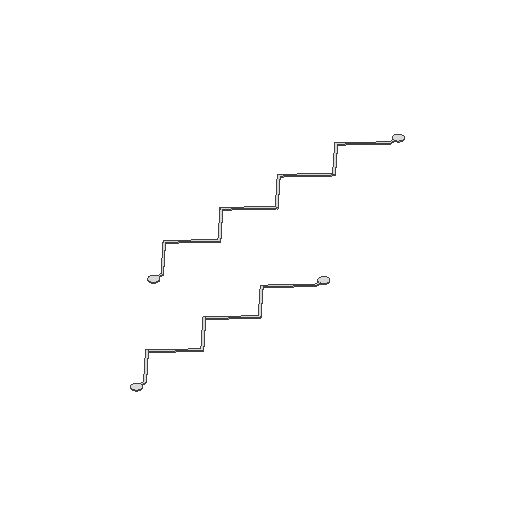
# Autodesk Inventor part: Serpentine
Saved by Autodesk Inventor 2025.4 (Build 294407000, 407)
## iProperties
Created: 2026-04-28
Part Number: Serpentine
Material: Generic
Document SubType Name: Modeling
Designer: gdira
Density: 1 g/cm^3
Appearance: Default
Author: gdira
Autodesk Inventor part; units mm, degrees
ref_plane "YZ Plane" through (0, 0, 0) normal (1, 0, 0) x (0, 1, 0)
ref_plane "XZ Plane" through (0, 0, 0) normal (0, 1, 0) x (-1, 0, 0)
ref_plane "XY Plane" through (0, 0, 0) normal (0, 0, 1) x (1, 0, 0)
sketch "Sketch1" plane through (0, 0, 0) normal (0, 1, 0) x (-1, 0, 0)
  line L0 (15, -130) -> (0, -130)
  line L1 (1.2651, -65) -> (15, -65)
  line L2 (1.2609, -97.5) -> (15, -97.5)
  line L3 (13.5021, -113.8888) -> (-0.2581, -115.1476)
  line L4 (15, -65) -> (1.2651, -65)
  line L5 (13.4695, -81.25) -> (-0.2581, -79.8524)
  line L6 (14.8669, 0) -> (0.0022, 0)
  line L7 (1.2651, -32.5) -> (15, -32.5)
  line L8 (13.4697, -16.25) -> (-0.2581, -14.8524)
  line L9 (13.4697, -48.75) -> (-0.2581, -50.1476)
  line L10 (0, -129.7127) -> (15, -113.75)
  line L11 (15, -113.75) -> (14.2713, -113.0652)
  line L12 (13.5021, -113.8888) -> (-1, -129.3217)
  line L13 (-1, -129.3217) -> (-0.9978, -129.3238)
  line L14 (15, -113.75) -> (0.6282, -98.1807)
  line L15 (-0.2652, -97.5) -> (-1, -98.1783)
  line L16 (-1, -98.1783) -> (13.5021, -113.8888)
  line L17 (14.2652, -114.4283) -> (15, -113.75)
  line L18 (-1, -98.1783) -> (14.102, -81.9307)
  line L19 (15, -81.25) -> (15.7325, -81.9308)
  line L20 (-0.2605, -98.8657) -> (-1, -98.1783)
  line L21 (15.7325, -81.9308) -> (0.6326, -65.6807)
  line L22 (-0.2652, -65) -> (-0.9978, -65.6807)
  line L23 (-0.9978, -65.6807) -> (14.102, -81.9307)
  line L24 (14.9999, -82.6115) -> (15.7325, -81.9308)
  line L25 (-0.9978, -65.6807) -> (14.1022, -49.4307)
  line L26 (15, -48.75) -> (15.7326, -49.4307)
  line L27 (15.7326, -49.4307) -> (0.6326, -65.6807)
  line L28 (-0.2652, -66.3614) -> (-0.9978, -65.6807)
  line L29 (15.7326, -49.4307) -> (0.6325, -33.1807)
  line L30 (-0.2652, -32.5) -> (-0.9978, -33.1807)
  line L31 (-0.9978, -33.1807) -> (14.1022, -49.4307)
  line L32 (15, -50.1114) -> (15.7326, -49.4307)
  line L33 (-0.9978, -33.1807) -> (14.1018, -16.9303)
  line L34 (14.8669, -16.3923) -> (15.5995, -17.073)
  line L35 (15.5995, -17.073) -> (0.6325, -33.1807)
  line L36 (-0.2652, -33.8614) -> (-0.9978, -33.1807)
  line L37 (15.5995, -17.073) -> (0.0022, -0.2878)
  line L38 (-0.9978, -0.6807) -> (14.1018, -16.9303)
  line L39 (15, -17.6114) -> (15.5995, -17.073)
  line L40 (-0.2652, -129.3217) -> (0, -129.3217)
  line L41 (0, -129.3217) -> (0, -131.8722)
  line L42 (-1, -131.8722) -> (-1, -129.3217)
  line L43 (0, -0.6807) -> (0.0022, -0.6807)
  line L44 (0.0022, -0.2878) -> (0.0022, 1.8698)
  line L45 (-0.9978, 1.8698) -> (-0.9978, -0.6807)
  arc A0 (0.0022, 1.8698) -> (-0.9978, 1.8698) centre (-0.4978, 4.3193) ccw
  arc A1 (-1, -131.8722) -> (0, -131.8722) centre (-0.5, -134.3217) ccw
  line L46 (0, -134.3217) -> (-0.2652, -134.3217)
  line L47 (-0.9978, -134.3217) -> (-1, -134.3217)
  line L48 (15.7325, -81.9308) -> (0.6282, -98.1807)
  line L49 (-0.2581, -98.8631) -> (-0.2605, -98.8657)
  line L50 (15, -82.6114) -> (15, -130)
  line L51 (-0.2652, -97.5) -> (-0.2652, -66.3614)
  line L52 (15, -50.1114) -> (15, -81.25)
  line L53 (-0.2652, -65) -> (-0.2652, -33.8614)
  line L54 (-0.2652, -32.5) -> (-0.2652, -1.4691)
  line L55 (14.8669, 0) -> (14.8669, -16.3923)
  line L56 (15, -17.6114) -> (15, -48.75)
  line L57 (0.0022, 4.3193) -> (0, 4.3193)
  line L58 (-0.2581, -128.5323) -> (-0.2581, -98.8631)
  line L59 (-33.8119, -38.9953) -> (-48.8119, -38.9953)
  line L60 (-47.5468, 26.0047) -> (-33.8119, 26.0047)
  line L61 (-47.5509, -6.4953) -> (-33.8119, -6.4953)
  line L62 (-35.3097, -22.8842) -> (-49.07, -24.1429)
  line L63 (-33.8119, 26.0047) -> (-47.5468, 26.0047)
  line L64 (-35.3424, 9.7546) -> (-49.07, 11.1522)
  line L65 (-35.3422, 42.2547) -> (-49.07, 40.8571)
  line L66 (-48.8119, -38.708) -> (-33.8119, -22.7453)
  line L67 (-33.8119, -22.7453) -> (-34.5406, -22.0605)
  line L68 (-35.3097, -22.8842) -> (-49.8119, -38.317)
  line L69 (-49.8119, -38.317) -> (-49.8096, -38.3191)
  line L70 (-33.8119, -22.7453) -> (-48.1836, -7.176)
  line L71 (-49.0771, -6.4953) -> (-49.8119, -7.1736)
  line L72 (-49.8119, -7.1736) -> (-35.3097, -22.8842)
  line L73 (-34.5467, -23.4236) -> (-33.8119, -22.7453)
  line L74 (-49.8119, -7.1736) -> (-34.7099, 9.0739)
  line L75 (-33.8119, 9.7547) -> (-33.0794, 9.0739)
  line L76 (-49.0724, -7.861) -> (-49.8119, -7.1736)
  line L77 (-33.0794, 9.0739) -> (-48.1793, 25.324)
  line L78 (-49.0771, 26.0047) -> (-49.8096, 25.324)
  line L79 (-49.8096, 25.324) -> (-34.7099, 9.0739)
  line L80 (-33.812, 8.3932) -> (-33.0794, 9.0739)
  line L81 (-49.8096, 25.324) -> (-34.7096, 41.574)
  line L82 (-33.8119, 42.2547) -> (-33.0793, 41.574)
  line L83 (-33.0793, 41.574) -> (-48.1793, 25.324)
  line L84 (-49.0771, 24.6433) -> (-49.8096, 25.324)
  line L85 (-33.0793, 41.574) -> (-48.1793, 57.824)
  line L86 (-49.8096, 57.8239) -> (-34.7096, 41.574)
  line L87 (-33.8119, 40.8932) -> (-33.0793, 41.574)
  line L88 (-49.0771, -38.317) -> (-48.8119, -38.317)
  line L89 (-48.8119, -38.317) -> (-48.8119, -40.8676)
  line L90 (-49.8119, -40.8676) -> (-49.8119, -38.317)
  arc A2 (-49.8119, -40.8676) -> (-48.8119, -40.8676) centre (-49.3119, -43.317) ccw
  line L91 (-48.8119, -43.317) -> (-49.0771, -43.317)
  line L92 (-49.8096, -43.3171) -> (-49.8119, -43.3171)
  line L93 (-33.0794, 9.0739) -> (-48.1836, -7.176)
  line L94 (-49.07, -7.8585) -> (-49.0724, -7.861)
  line L95 (-33.8119, 8.3932) -> (-33.8119, -38.9953)
  line L96 (-49.0771, -6.4953) -> (-49.0771, 24.6433)
  line L97 (-33.8119, 40.8932) -> (-33.8119, 9.7547)
  line L98 (-49.0771, 26.0047) -> (-49.0771, 57.1433)
  line L99 (-33.8119, 73.3932) -> (-33.8119, 42.2547)
  line L100 (-49.07, -37.5276) -> (-49.07, -7.8585)
  line L101 (-49.0771, 57.1433) -> (-48.8119, 57.1433)
  line L102 (-48.0771, 57.1433) -> (-48.0771, 62.1433)
  line L103 (-48.0771, 62.1433) -> (-49.0771, 62.1433)
  line L104 (-49.0771, 62.1433) -> (-49.0771, 57.1433)
  circle A3 centre (-48.5771, 62.1433) radius 2.5
  point P0 (0, 0)
  point P1 (15, -16.25)
  point P2 (15, -82.7188)
  point P3 (15, -81.1426)
  point P4 (15, -50.2191)
  point P5 (15, -48.6424)
  point P6 (15, -17.7181)
  point P7 (14.8669, -16.2846)
  point P8 (-0.2652, -32.3923)
  point P9 (-0.2652, -33.9691)
  point P10 (-0.2652, -64.8923)
  point P11 (-0.2652, -66.469)
  point P12 (-0.2652, -97.3877)
  point P13 (-0.2581, -98.982)
  point P14 (-33.8119, 8.2858)
  point P15 (-33.8119, 9.8621)
  point P16 (-33.8119, 40.7856)
  point P17 (-33.8119, 42.3623)
  point P18 (-48.0771, 57.7139)
  point P19 (-48.0771, 59.6938)
  point P20 (-49.0771, 59.6938)
  point P21 (-49.0771, 57.0356)
  point P22 (-49.0771, 26.1123)
  point P23 (-49.0771, 24.5356)
  point P24 (-49.0771, -6.3831)
  point P25 (-49.07, -7.9773)
  point P26 (-0.4978, 6.8193)
  point P27 (-0.5, -136.8217)
  point P28 (-49.3119, -45.817)
  dimension "d0" = 15
  dimension "d2" = 1
  dimension "d3" = 1
  dimension "d4" = 1
  dimension "d5" = 1
  dimension "d6" = 1
  dimension "d7" = 1
  dimension "d8" = 1
  dimension "d10" = 1
  dimension "d11" = 5
  dimension "d12" = 1
  dimension "d13" = 5
  dimension "d14" = 5
  dimension "d15" = 5
  dimension "d18" = 15
  dimension "d19" = 1
  dimension "d20" = 1
  dimension "d21" = 1
  dimension "d22" = 1
  dimension "d23" = 1
  dimension "d26" = 1
  dimension "d27" = 5
  dimension "d31" = 5
  dimension "d32" = 1
  dimension "d33" = 5
  dimension "d34" = 5
  dimension "d35" = 143.641
  dimension "d36" = 107.9603
  constraints: 210 end point, 63 parallel, 34 point on line, 32 perpendicular, 12 symmetric about line, 9 point on circle, 4 centre point, 1 horizontal, 1 midpoint
  measures "d0" distance of L0.start L0.end
  measures "d2" distance of L11.end L10.end
  measures "d3" distance of L15.end L15.start
  measures "d4" distance of L19.start L19.end
  measures "d5" distance of L22.end L22.start
  measures "d6" distance of L26.start L26.end
  measures "d7" distance of L30.end L30.start
  measures "d8" distance of L34.start L34.end
  measures "d10" distance of L12.end L40.end
  measures "d11" distance of L40.end L46.start
  measures "d12" distance of L38.start L43.end
  measures "d13" distance of L57.start L43.end
  measures "d14" diameter of A0
  measures "d15" diameter of A1
  measures "d18" distance of L59.start L59.end
  measures "d19" distance of L67.end L66.end
  measures "d20" distance of L76.end L71.start
  measures "d21" distance of L97.end L75.end
  measures "d22" distance of L78.end L78.start
  measures "d23" distance of L82.start L83.start
  measures "d26" distance of L69.start L88.end
  measures "d27" distance of L88.end L91.start
  measures "d31" diameter of A2
  measures "d32" distance of L98.end L102.start
  measures "d33" distance of L102.end L102.start
  measures "d34" diameter of A3
  measures "d35" distance of point (-0.498, 6.819) point (-0.5, -136.822)
  measures "d36" vertical distance of A3.centre point (-49.312, -45.817)
extrude "Extrusion1" add sketch "Sketch1" along normal blind 0.5 contours L41 A1 L42 L12 L16 L58 L49 L20 L15 L51 L18 L23 L28 L22 L53 L25 L31 L36 L30 L54 L33 L38 L45 A0 L44 L37 L55 L34 L39 L56 L35 L29 L26 L32 L52 L27 L21 L19 L24 L50 L48 L14 L10 | L89 A2 L90 L68 L72 L100 L94 L76 L71 L96 L74 L79 L84 L78 L98 L81 L86 L104 A3 L102 L85 L99 L82 L87 L97 L83 L77 L75 L80 L95 L93 L70 L66 | A3 L104 L103 L102 | L102 L103 L104 A3
body "Solid1"
